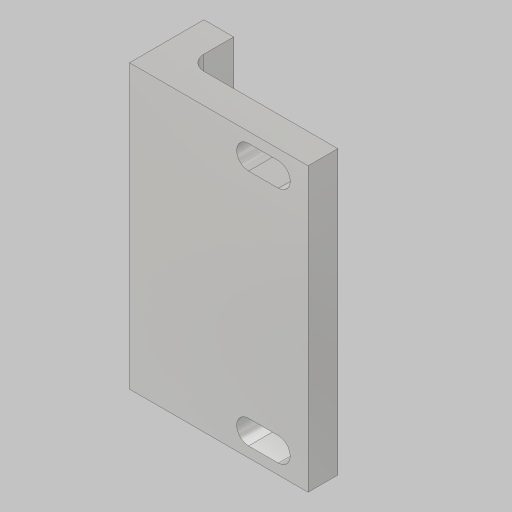
# Autodesk Inventor part: HS-001
Saved by Autodesk Inventor 2023.5 (Build 275446000, 446)
## iProperties
Created: 2025-02-22
Part Number: HS-001
Material: Aluminum 6061
Document SubType Name: Modeling
Designer: slick
Density: 2.7 g/cm^3
Appearance: Aluminum - Polished
Author: slick
Autodesk Inventor part; units mm, degrees
ref_plane "YZ Plane" through (0, 0, 0) normal (1, 0, 0) x (0, 1, 0)
ref_plane "XZ Plane" through (0, 0, 0) normal (0, 1, 0) x (-1, 0, 0)
ref_plane "XY Plane" through (0, 0, 0) normal (0, 0, 1) x (1, 0, 0)
sketch "Sketch1" plane through (0, 0, 0) normal (0, 1, 0) x (-1, 0, 0)
  line L0 (0, 0) -> (0, -6.35)
  line L1 (0, -6.35) -> (31.75, -6.35)
  line L2 (31.75, -6.35) -> (31.75, -15.875)
  line L3 (31.75, -15.875) -> (38.1, -15.875)
  line L4 (38.1, -15.875) -> (38.1, 0)
  line L5 (38.1, 0) -> (0, 0)
  dimension "d0" = 6.35
  dimension "d1" = 38.1
  dimension "d2" = 15.875
  constraints: 12 end point, 6 perpendicular, 1 vertical
  measures "d0" distance of L0.start L0.end
  measures "d1" distance of L4.end L0.start
  measures "d2" distance of L3.end L4.end
extrude "Extrusion1" add sketch "Sketch1" along normal blind 60.325
sketch "Sketch2" plane through (-38.1, 0, 0) normal (0, 0, 1) x (1, 0, 0)
  line L0 (31.75, 4.7625) -> (31.75, 55.5625) construction
  line L1 (38.1, 0) -> (38.1, 60.325) construction
  line L2 (25.4, 4.7625) -> (31.75, 4.7625) construction
  line L3 (25.4, 2.2098) -> (31.75, 2.2098)
  line L4 (31.75, 7.3152) -> (25.4, 7.3152)
  arc A0 (25.4, 7.3152) -> (25.4, 2.2098) centre (25.4, 4.7625) ccw
  arc A1 (31.75, 2.2098) -> (31.75, 7.3152) centre (31.75, 4.7625) ccw
  line L5 (25.4, 55.5625) -> (31.75, 55.5625) construction
  line L6 (25.4, 53.0098) -> (31.75, 53.0098)
  line L7 (31.75, 58.1152) -> (25.4, 58.1152)
  arc A2 (25.4, 58.1152) -> (25.4, 53.0098) centre (25.4, 55.5625) ccw
  arc A3 (31.75, 53.0098) -> (31.75, 58.1152) centre (31.75, 55.5625) ccw
  point P0 (31.75, 30.1625)
  point P1 (38.1, 30.1625)
  point P2 (28.575, 4.7625)
  point P3 (28.575, 55.5625)
  dimension "d5" = 50.8
  dimension "d6" = 6.35
  dimension "d24" = 5.1054
  dimension "d25" = 6.35
  constraints: 18 end point, 8 point on circle, 8 tangent, 4 centre point, 4 midpoint, 3 horizontal alignment, 3 vertical alignment, 2 horizontal, 2 parallel, 1 equal radius, 1 vertical
  measures "d5" distance of L0.start L0.end
  measures "d6" distance between parallel lines of L1 L0
  measures "d24" distance between parallel lines of L4 L3
  measures "d25" distance of L2.start L0.start
sketch "Sketch3" plane through (-38.1, 0, -15.875) normal (-1, 0, 0) x (0, 0, 1)
  line L0 (7.62, 46.1625) -> (7.62, 14.1625) construction
  line L1 (0, 0) -> (0, 60.325) construction
  line L2 (0, 60.325) -> (15.875, 60.325) construction
  line L3 (15.875, 0) -> (15.875, 60.325) construction
  point P0 (7.62, 30.1625)
  point P1 (0, 30.1625)
  point P2 (7.9375, 60.325)
  dimension "d14" = 32
  dimension "d23" = 8.255
  constraints: 3 midpoint, 2 end point, 1 horizontal alignment, 1 vertical
  measures "d14" distance of L0.start L0.end
  measures "d23" distance between parallel lines of L3 L0
hole "Hole2" at (-38.1, 46.1625, -8.255) at (-38.1, 14.1625, -8.255) direction (1, 0, 0) diameter 2.6416 depth 19.05 tip angle 118 thread size "6-32 UNC" class "2B" standard "ANSI Unified Screw Threads"
extrude "Extrusion2" cut sketch "Sketch2" against normal blind 25.4
fillet "Fillet2" radius 3.175 1 edges at (-31.75, 30.1625, -6.35)
body "Solid1"
